Autodesk Fusion 360 part; units mm, degrees
(part 4 of 6)
  spline S229 degree 3 poles (64.9154, 36.2009) (64.8548, 36.2983) (64.7292, 36.5001) (64.6717, 36.7309) (64.642, 36.8503) knots 0 0 0 0 0.034206 0.07085 0.07085 0.07085 0.07085
  spline S230 degree 3 poles (64.642, 36.8503) (64.6279, 36.962) (64.5921, 37.2456) (64.5928, 37.5315) (64.5931, 37.7048) knots 0 0 0 0 0.033768 0.085663 0.085663 0.085663 0.085663
  line L165 (64.5931, 37.7048) -> (64.5931, 40.8932)
  line L166 (64.5931, 40.8932) -> (65.472, 40.8932)
  line L167 (65.472, 40.8932) -> (65.472, 37.7389)
  spline S231 degree 3 poles (65.472, 37.7389) (65.4729, 37.5814) (65.4743, 37.309) (65.5449, 37.0464) (65.5746, 36.9357) knots 0 0 0 0 0.047006 0.081267 0.081267 0.081267 0.081267
  spline S232 degree 3 poles (65.5746, 36.9357) (65.6162, 36.851) (65.7009, 36.6784) (65.8582, 36.5674) (65.9384, 36.5109) knots 0 0 0 0 0.027833 0.056732 0.056732 0.056732 0.056732
  spline S233 degree 3 poles (65.9384, 36.5109) (66.0312, 36.4646) (66.2241, 36.3686) (66.4395, 36.3578) (66.5511, 36.3522) knots 0 0 0 0 0.030776 0.063912 0.063912 0.063912 0.063912
  spline S234 degree 3 poles (66.5511, 36.3522) (66.7312, 36.3665) (67.0878, 36.3947) (67.3772, 36.6047) (67.5204, 36.7087) knots 0 0 0 0 0.053061 0.105073 0.105073 0.105073 0.105073
  spline S235 degree 3 poles (67.5204, 36.7087) (67.6385, 36.8753) (67.9223, 37.2758) (67.926, 37.7716) (67.9281, 38.0612) knots 0 0 0 0 0.060011 0.144248 0.144248 0.144248 0.144248
  line L168 (67.9281, 38.0612) -> (67.9281, 40.8932)
  line L169 (67.9281, 40.8932) -> (68.807, 40.8932)
  line L170 (56.9174, 39.2233) -> (56.0092, 39.3356)
  spline S236 degree 3 poles (56.0092, 39.3356) (56.0926, 39.5834) (56.2541, 40.0629) (56.6255, 40.4055) (56.8051, 40.571) knots 0 0 0 0 0.077034 0.149075 0.149075 0.149075 0.149075
  spline S237 degree 3 poles (56.8051, 40.571) (57.02, 40.699) (57.4764, 40.9709) (58.0081, 40.9968) (58.2894, 41.0104) knots 0 0 0 0 0.073917 0.156923 0.156923 0.156923 0.156923
  spline S238 degree 3 poles (58.2894, 41.0104) (58.6434, 40.987) (59.3202, 40.9421) (59.8438, 40.514) (60.0936, 40.3097) knots 0 0 0 0 0.103483 0.197891 0.197891 0.197891 0.197891
  spline S239 degree 3 poles (60.0936, 40.3097) (60.2877, 40.039) (60.7071, 39.454) (60.7416, 38.7321) (60.7601, 38.3444) knots 0 0 0 0 0.097893 0.211487 0.211487 0.211487 0.211487
  spline S240 degree 3 poles (60.7601, 38.3444) (60.7418, 37.9438) (60.7079, 37.2003) (60.2825, 36.5932) (60.0863, 36.3132) knots 0 0 0 0 0.117426 0.217964 0.217964 0.217964 0.217964
  spline S241 degree 3 poles (60.0863, 36.3132) (59.8409, 36.1024) (59.3383, 35.6707) (58.6768, 35.6177) (58.3383, 35.5905) knots 0 0 0 0 0.094484 0.193557 0.193557 0.193557 0.193557
  spline S242 degree 3 poles (58.3383, 35.5905) (58.0098, 35.6175) (57.3662, 35.6704) (56.8781, 36.092) (56.639, 36.2985) knots 0 0 0 0 0.096126 0.18838 0.18838 0.18838 0.18838
  spline S243 degree 3 poles (56.639, 36.2985) (56.4471, 36.5731) (56.0307, 37.1688) (55.9977, 37.8977) (55.9799, 38.2907) knots 0 0 0 0 0.098509 0.213708 0.213708 0.213708 0.213708
  spline S244 degree 3 poles (55.9799, 38.2907) (55.9802, 38.3233) (55.9809, 38.4014) (55.9833, 38.4795) (55.9847, 38.5251) knots 0 0 0 0 0.009766 0.023443 0.023443 0.023443 0.023443
  line L171 (55.9847, 38.5251) -> (59.8519, 38.5251)
  spline S245 degree 3 poles (59.8519, 38.5251) (59.8265, 38.7854) (59.7797, 39.2658) (59.4977, 39.6553) (59.3685, 39.8337) knots 0 0 0 0 0.076825 0.141746 0.141746 0.141746 0.141746
  spline S246 degree 3 poles (59.3685, 39.8337) (59.2137, 39.9661) (58.9013, 40.2335) (58.4914, 40.2696) (58.2845, 40.2878) knots 0 0 0 0 0.059532 0.120175 0.120175 0.120175 0.120175
  spline S247 degree 3 poles (58.2845, 40.2878) (58.1314, 40.2787) (57.8353, 40.2612) (57.5818, 40.1079) (57.4593, 40.0339) knots 0 0 0 0 0.045247 0.087501 0.087501 0.087501 0.087501
  spline S248 degree 3 poles (57.4593, 40.0339) (57.349, 39.9297) (57.1072, 39.7015) (56.9842, 39.3917) (56.9174, 39.2233) knots 0 0 0 0 0.045001 0.098557 0.098557 0.098557 0.098557
  line L172 (46.0238, 40.8932) -> (46.0238, 35.7077)
  line L173 (46.0238, 35.7077) -> (45.2328, 35.7077)
  line L174 (45.2328, 35.7077) -> (45.2328, 36.4938)
  spline S249 degree 3 poles (45.2328, 36.4938) (45.1447, 36.3341) (44.9948, 36.0624) (44.7674, 35.8527) (44.6737, 35.7663) knots 0 0 0 0 0.05425 0.092273 0.092273 0.092273 0.092273
  spline S250 degree 3 poles (44.6737, 35.7663) (44.5863, 35.715) (44.4119, 35.6128) (44.2103, 35.5979) (44.1097, 35.5905) knots 0 0 0 0 0.029972 0.059777 0.059777 0.059777 0.059777
  spline S251 degree 3 poles (44.1097, 35.5905) (43.9575, 35.6045) (43.6366, 35.6341) (43.3546, 35.7912) (43.2064, 35.8737) knots 0 0 0 0 0.045356 0.095599 0.095599 0.095599 0.095599
  line L175 (43.2064, 35.8737) -> (43.5092, 36.6891)
  spline S252 degree 3 poles (43.5092, 36.6891) (43.6143, 36.6336) (43.8166, 36.5268) (44.0443, 36.5078) (44.1537, 36.4987) knots 0 0 0 0 0.03525 0.067826 0.067826 0.067826 0.067826
  spline S253 degree 3 poles (44.1537, 36.4987) (44.2473, 36.5059) (44.4343, 36.5203) (44.5923, 36.6215) (44.6713, 36.672) knots 0 0 0 0 0.027685 0.055345 0.055345 0.055345 0.055345
  spline S254 degree 3 poles (44.6713, 36.672) (44.7427, 36.7369) (44.8902, 36.8708) (44.9616, 37.057) (44.9984, 37.153) knots 0 0 0 0 0.028537 0.058895 0.058895 0.058895 0.058895
  spline S255 degree 3 poles (44.9984, 37.153) (45.0411, 37.3157) (45.1294, 37.6518) (45.1396, 37.9992) (45.1449, 38.1784) knots 0 0 0 0 0.050287 0.103879 0.103879 0.103879 0.103879
  line L176 (45.1449, 38.1784) -> (45.1449, 40.8932)
  line L177 (45.1449, 40.8932) -> (46.0238, 40.8932)
  line L178 (42.6791, 40.8932) -> (42.6791, 35.7077)
  line L179 (42.6791, 35.7077) -> (41.8002, 35.7077)
  line L180 (41.8002, 35.7077) -> (41.8002, 40.8932)
  line L181 (41.8002, 40.8932) -> (42.6791, 40.8932)
  line L182 (40.8138, 39.3454) -> (39.9447, 39.2087)
  spline S256 degree 3 poles (39.9447, 39.2087) (39.9126, 39.3698) (39.8517, 39.6759) (39.6381, 39.9023) (39.537, 40.0095) knots 0 0 0 0 0.048178 0.091492 0.091492 0.091492 0.091492
  spline S257 degree 3 poles (39.537, 40.0095) (39.4069, 40.0905) (39.1219, 40.268) (38.785, 40.2808) (38.6019, 40.2878) knots 0 0 0 0 0.045208 0.099065 0.099065 0.099065 0.099065
  spline S258 degree 3 poles (38.6019, 40.2878) (38.4213, 40.2836) (38.0995, 40.2762) (37.8242, 40.1128) (37.7035, 40.0412) knots 0 0 0 0 0.053093 0.094556 0.094556 0.094556 0.094556
  spline S259 degree 3 poles (37.7035, 40.0412) (37.6181, 39.9579) (37.454, 39.7979) (37.4246, 39.5712) (37.4105, 39.4626) knots 0 0 0 0 0.034652 0.06657 0.06657 0.06657 0.06657
  spline S260 degree 3 poles (37.4105, 39.4626) (37.4218, 39.3682) (37.4447, 39.1773) (37.5938, 39.0555) (37.6693, 38.9938) knots 0 0 0 0 0.027386 0.055446 0.055446 0.055446 0.055446
  spline S261 degree 3 poles (37.6693, 38.9938) (37.7734, 38.9471) (38.0623, 38.8174) (38.3706, 38.7433) (38.5677, 38.696) knots 0 0 0 0 0.034189 0.094822 0.094822 0.094822 0.094822
  spline S262 degree 3 poles (38.5677, 38.696) (38.8428, 38.6271) (39.2983, 38.513) (39.7351, 38.3415) (39.9081, 38.2736) knots 0 0 0 0 0.084955 0.140654 0.140654 0.140654 0.140654
  spline S263 degree 3 poles (39.9081, 38.2736) (40.024, 38.2102) (40.2491, 38.0871) (40.4009, 37.8806) (40.4745, 37.7804) knots 0 0 0 0 0.039108 0.075916 0.075916 0.075916 0.075916
  spline S264 degree 3 poles (40.4745, 37.7804) (40.5307, 37.6722) (40.6442, 37.454) (40.6596, 37.2084) (40.6674, 37.0846) knots 0 0 0 0 0.036161 0.072917 0.072917 0.072917 0.072917
  spline S265 degree 3 poles (40.6674, 37.0846) (40.661, 36.9717) (40.6483, 36.7476) (40.5549, 36.5437) (40.5087, 36.4426) knots 0 0 0 0 0.033621 0.066662 0.066662 0.066662 0.066662
  spline S266 degree 3 poles (40.5087, 36.4426) (40.451, 36.3482) (40.3355, 36.1595) (40.1629, 36.0211) (40.0765, 35.9518) knots 0 0 0 0 0.032897 0.065829 0.065829 0.065829 0.065829
  spline S267 degree 3 poles (40.0765, 35.9518) (39.9973, 35.902) (39.8224, 35.792) (39.6253, 35.7296) (39.5175, 35.6955) knots 0 0 0 0 0.027973 0.061727 0.061727 0.061727 0.061727
  spline S268 degree 3 poles (39.5175, 35.6955) (39.3958, 35.6649) (39.1466, 35.6022) (38.8897, 35.5945) (38.7582, 35.5905) knots 0 0 0 0 0.037518 0.076851 0.076851 0.076851 0.076851
  spline S269 degree 3 poles (38.7582, 35.5905) (38.5656, 35.5961) (38.2002, 35.6067) (37.8514, 35.7151) (37.6864, 35.7663) knots 0 0 0 0 0.05748 0.109059 0.109059 0.109059 0.109059
  spline S270 degree 3 poles (37.6864, 35.7663) (37.546, 35.8258) (37.2846, 35.9365) (37.0936, 36.1456) (37.0052, 36.2424) knots 0 0 0 0 0.045124 0.083974 0.083974 0.083974 0.083974
  spline S271 degree 3 poles (37.0052, 36.2424) (36.9368, 36.3568) (36.7878, 36.6059) (36.7325, 36.8913) (36.7025, 37.0456) knots 0 0 0 0 0.039698 0.086419 0.086419 0.086419 0.086419
  line L183 (36.7025, 37.0456) -> (37.5619, 37.1628)
  spline S272 degree 3 poles (37.5619, 37.1628) (37.5891, 37.038) (37.6417, 36.7963) (37.8166, 36.622) (37.9012, 36.5378) knots 0 0 0 0 0.037427 0.072477 0.072477 0.072477 0.072477
  spline S273 degree 3 poles (37.9012, 36.5378) (38.0114, 36.4724) (38.2549, 36.3279) (38.5391, 36.3184) (38.6947, 36.3132) knots 0 0 0 0 0.037832 0.083649 0.083649 0.083649 0.083649
  spline S274 degree 3 poles (38.6947, 36.3132) (38.8716, 36.3146) (39.1763, 36.317) (39.4459, 36.4553) (39.559, 36.5134) knots 0 0 0 0 0.052121 0.089788 0.089788 0.089788 0.089788
  spline S275 degree 3 poles (39.559, 36.5134) (39.6344, 36.5801) (39.777, 36.7062) (39.8047, 36.8937) (39.8177, 36.9821) knots 0 0 0 0 0.029135 0.0551 0.0551 0.0551 0.0551
  spline S276 degree 3 poles (39.8177, 36.9821) (39.8132, 37.0378) (39.804, 37.1496) (39.7417, 37.2429) (39.7103, 37.2897) knots 0 0 0 0 0.016456 0.033067 0.033067 0.033067 0.033067
  spline S277 degree 3 poles (39.7103, 37.2897) (39.6666, 37.336) (39.5708, 37.4373) (39.4429, 37.4935) (39.3734, 37.5241) knots 0 0 0 0 0.018913 0.04141 0.04141 0.04141 0.04141
  spline S278 degree 3 poles (39.3734, 37.5241) (39.2869, 37.5514) (39.0299, 37.6324) (38.7696, 37.7023) (38.597, 37.7487) knots 0 0 0 0 0.027221 0.080828 0.080828 0.080828 0.080828
  spline S279 degree 3 poles (38.597, 37.7487) (38.3316, 37.8192) (37.8917, 37.936) (37.465, 38.0939) (37.2958, 38.1564) knots 0 0 0 0 0.082338 0.13643 0.13643 0.13643 0.13643
  spline S280 degree 3 poles (37.2958, 38.1564) (37.1803, 38.2141) (36.9546, 38.327) (36.7951, 38.5224) (36.7172, 38.6179) knots 0 0 0 0 0.038228 0.07476 0.07476 0.07476 0.07476
  spline S281 degree 3 poles (36.7172, 38.6179) (36.656, 38.7285) (36.5267, 38.962) (36.5139, 39.2292) (36.5072, 39.3698) knots 0 0 0 0 0.037411 0.079003 0.079003 0.079003 0.079003
  spline S282 degree 3 poles (36.5072, 39.3698) (36.5185, 39.5151) (36.5415, 39.8102) (36.6888, 40.0671) (36.7635, 40.1974) knots 0 0 0 0 0.043142 0.087613 0.087613 0.087613 0.087613
  spline S283 degree 3 poles (36.7635, 40.1974) (36.861, 40.3206) (37.0627, 40.5755) (37.3532, 40.7222) (37.5033, 40.798) knots 0 0 0 0 0.046534 0.096306 0.096306 0.096306 0.096306
  spline S284 degree 3 poles (37.5033, 40.798) (37.6733, 40.86) (38.0264, 40.9886) (38.4021, 41.003) (38.597, 41.0104) knots 0 0 0 0 0.053921 0.112025 0.112025 0.112025 0.112025
  spline S285 degree 3 poles (38.597, 41.0104) (38.9016, 41.0018) (39.4515, 40.9863) (39.9259, 40.7126) (40.1376, 40.5905) knots 0 0 0 0 0.089667 0.161897 0.161897 0.161897 0.161897
  spline S286 degree 3 poles (40.1376, 40.5905) (40.2994, 40.4263) (40.6433, 40.0773) (40.7548, 39.5988) (40.8138, 39.3454) knots 0 0 0 0 0.067824 0.14416 0.14416 0.14416 0.14416
  line L184 (42.6791, 34.7458) -> (42.6791, 33.735)
  line L185 (42.6791, 33.735) -> (41.8002, 33.735)
  line L186 (41.8002, 33.735) -> (41.8002, 34.7458)
  line L187 (41.8002, 34.7458) -> (42.6791, 34.7458)
  line L188 (51.5756, 42.8805) -> (51.5756, 35.7077)
  line L189 (51.5756, 35.7077) -> (50.7748, 35.7077)
  line L190 (50.7748, 35.7077) -> (50.7748, 36.3815)
  spline S287 degree 3 poles (50.7748, 36.3815) (50.6803, 36.2596) (50.4996, 36.0265) (50.2528, 35.8652) (50.1351, 35.7883) knots 0 0 0 0 0.045899 0.087785 0.087785 0.087785 0.087785
  spline S288 degree 3 poles (50.1351, 35.7883) (50.0056, 35.7306) (49.7309, 35.6084) (49.43, 35.5967) (49.2709, 35.5905) knots 0 0 0 0 0.042126 0.089382 0.089382 0.089382 0.089382
  spline S289 degree 3 poles (49.2709, 35.5905) (49.058, 35.6035) (48.6412, 35.6288) (48.2771, 35.8326) (48.099, 35.9323) knots 0 0 0 0 0.063081 0.123479 0.123479 0.123479 0.123479
  spline S290 degree 3 poles (48.099, 35.9323) (47.9391, 36.0605) (47.6107, 36.3236) (47.4268, 36.7024) (47.3324, 36.8967) knots 0 0 0 0 0.060684 0.124573 0.124573 0.124573 0.124573
  spline S291 degree 3 poles (47.3324, 36.8967) (47.2569, 37.1121) (47.1022, 37.5538) (47.0833, 38.0217) (47.0736, 38.2614) knots 0 0 0 0 0.068072 0.139594 0.139594 0.139594 0.139594
  spline S292 degree 3 poles (47.0736, 38.2614) (47.0838, 38.5162) (47.1036, 39.0093) (47.276, 39.4713) (47.3593, 39.6945) knots 0 0 0 0 0.075959 0.146956 0.146956 0.146956 0.146956
  spline S293 degree 3 poles (47.3593, 39.6945) (47.4631, 39.8932) (47.6662, 40.2816) (48.0176, 40.5432) (48.1893, 40.6711) knots 0 0 0 0 0.066289 0.129644 0.129644 0.129644 0.129644
  spline S294 degree 3 poles (48.1893, 40.6711) (48.3713, 40.77) (48.7291, 40.9646) (49.135, 40.9953) (49.3343, 41.0104) knots 0 0 0 0 0.061373 0.120639 0.120639 0.120639 0.120639
  spline S295 degree 3 poles (49.3343, 41.0104) (49.4754, 41.0036) (49.7498, 40.9903) (50.0009, 40.879) (50.1229, 40.8249) knots 0 0 0 0 0.041944 0.081634 0.081634 0.081634 0.081634
  spline S296 degree 3 poles (50.1229, 40.8249) (50.2332, 40.7601) (50.4488, 40.6335) (50.6153, 40.4471) (50.6967, 40.3561) knots 0 0 0 0 0.038106 0.074489 0.074489 0.074489 0.074489
  line L191 (50.6967, 40.3561) -> (50.6967, 42.8805)
  line L192 (50.6967, 42.8805) -> (51.5756, 42.8805)
  line L193 (27.483, 42.2234) -> (-5.7946, 42.2234) construction
  line L194 (-5.7946, 42.2234) -> (-5.7946, 34.7234) construction
  line L195 (-5.7946, 34.7234) -> (27.483, 34.7234) construction
  line L196 (27.483, 34.7234) -> (27.483, 42.2234) construction
  text T0 "Enterprise" font "Arial" height 7.5 align ink ink in box 0 x 0 at (27.483, 42.2234) x (-1, 0) y (0, -1) spacing 1 height is em
  constraint perpendicular L193 L194
  constraint parallel L193 L195
  constraint parallel L194 L196
extrude "Extrude22" add sketch "Sketch23" along normal blind 2 text T0 bodies 15
sketch "Sketch24" plane through (0, 3, 0) normal (0, 1, 0) x (-1, 0, 0)
  line L0 (27.473, 40.7129) -> (27.473, 35.3442)
  line L1 (27.473, 35.3442) -> (23.5912, 35.3442)
  line L2 (23.5912, 35.3442) -> (23.5912, 35.9778)
  line L3 (23.5912, 35.9778) -> (26.7626, 35.9778)
  line L4 (26.7626, 35.9778) -> (26.7626, 37.6221)
  line L5 (26.7626, 37.6221) -> (23.7926, 37.6221)
  line L6 (23.7926, 37.6221) -> (23.7926, 38.2519)
  line L7 (23.7926, 38.2519) -> (26.7626, 38.2519)
  line L8 (26.7626, 38.2519) -> (26.7626, 40.0793)
  line L9 (26.7626, 40.0793) -> (23.4667, 40.0793)
  line L10 (23.4667, 40.0793) -> (23.4667, 40.7129)
  line L11 (23.4667, 40.7129) -> (27.473, 40.7129)
  line L12 (16.9591, 40.1233) -> (16.8639, 40.7056)
  spline S0 degree 3 poles (16.8639, 40.7056) (16.9515, 40.7226) (17.1161, 40.7547) (17.2836, 40.7611) (17.3619, 40.7641) knots 0 0 0 0 0.026731 0.050214 0.050214 0.050214 0.050214
  spline S1 degree 3 poles (17.3619, 40.7641) (17.4698, 40.7621) (17.6628, 40.7584) (17.8403, 40.6836) (17.9186, 40.6506) knots 0 0 0 0 0.031987 0.057267 0.057267 0.057267 0.057267
  spline S2 degree 3 poles (17.9186, 40.6506) (17.9791, 40.6109) (18.0964, 40.534) (18.1641, 40.4114) (18.1969, 40.3522) knots 0 0 0 0 0.021363 0.04136 0.04136 0.04136 0.04136
  spline S3 degree 3 poles (18.1969, 40.3522) (18.2201, 40.2569) (18.282, 40.0018) (18.2792, 39.7387) (18.2775, 39.574) knots 0 0 0 0 0.029331 0.07849 0.07849 0.07849 0.07849
  line L13 (18.2775, 39.574) -> (18.2775, 37.3364)
  line L14 (18.2775, 37.3364) -> (18.7609, 37.3364)
  line L15 (18.7609, 37.3364) -> (18.7609, 36.8237)
  line L16 (18.7609, 36.8237) -> (18.2775, 36.8237)
  line L17 (18.2775, 36.8237) -> (18.2775, 35.8606)
  line L18 (18.2775, 35.8606) -> (17.622, 35.4651)
  line L19 (17.622, 35.4651) -> (17.622, 36.8237)
  line L20 (17.622, 36.8237) -> (16.9591, 36.8237)
  line L21 (16.9591, 36.8237) -> (16.9591, 37.3364)
  line L22 (16.9591, 37.3364) -> (17.622, 37.3364)
  line L23 (17.622, 37.3364) -> (17.622, 39.6106)
  spline S4 degree 3 poles (17.622, 39.6106) (17.6229, 39.6882) (17.6245, 39.8106) (17.5971, 39.9296) (17.5872, 39.9731) knots 0 0 0 0 0.023179 0.036529 0.036529 0.036529 0.036529
  spline S5 degree 3 poles (17.5872, 39.9731) (17.5736, 39.9987) (17.546, 40.0505) (17.498, 40.0842) (17.4736, 40.1013) knots 0 0 0 0 0.00856 0.01734 0.01734 0.01734 0.01734
  spline S6 degree 3 poles (17.4736, 40.1013) (17.4422, 40.1151) (17.3707, 40.1466) (17.2923, 40.1481) (17.2484, 40.1489) knots 0 0 0 0 0.010212 0.023221 0.023221 0.023221 0.023221
  spline S7 degree 3 poles (17.2484, 40.1489) (17.2059, 40.1474) (17.1091, 40.144) (17.013, 40.1307) (16.9591, 40.1233) knots 0 0 0 0 0.012742 0.02906 0.02906 0.02906 0.02906
  line L24 (12.1508, 40.7129) -> (12.1508, 36.8237)
  line L25 (12.1508, 36.8237) -> (11.5575, 36.8237)
  line L26 (11.5575, 36.8237) -> (11.5575, 37.4133)
  spline S8 degree 3 poles (11.5575, 37.4133) (11.4914, 37.2935) (11.379, 37.0898) (11.2085, 36.9325) (11.1382, 36.8677) knots 0 0 0 0 0.040688 0.069205 0.069205 0.069205 0.069205
  spline S9 degree 3 poles (11.1382, 36.8677) (11.0726, 36.8292) (10.9418, 36.7525) (10.7906, 36.7414) (10.7152, 36.7358) knots 0 0 0 0 0.022479 0.044833 0.044833 0.044833 0.044833
  spline S10 degree 3 poles (10.7152, 36.7358) (10.601, 36.7464) (10.3603, 36.7685) (10.1489, 36.8863) (10.0377, 36.9482) knots 0 0 0 0 0.034017 0.071699 0.071699 0.071699 0.071699
  line L27 (10.0377, 36.9482) -> (10.2648, 37.5598)
  spline S11 degree 3 poles (10.2648, 37.5598) (10.3436, 37.5182) (10.4953, 37.438) (10.6661, 37.4238) (10.7482, 37.417) knots 0 0 0 0 0.026437 0.050869 0.050869 0.050869 0.050869
  spline S12 degree 3 poles (10.7482, 37.417) (10.8184, 37.4224) (10.9586, 37.4332) (11.0771, 37.5091) (11.1364, 37.547) knots 0 0 0 0 0.020764 0.041509 0.041509 0.041509 0.041509
  spline S13 degree 3 poles (11.1364, 37.547) (11.19, 37.5956) (11.3006, 37.6961) (11.3541, 37.8357) (11.3817, 37.9077) knots 0 0 0 0 0.021403 0.044172 0.044172 0.044172 0.044172
  spline S14 degree 3 poles (11.3817, 37.9077) (11.4138, 38.0297) (11.4799, 38.2818) (11.4876, 38.5423) (11.4916, 38.6767) knots 0 0 0 0 0.037715 0.077909 0.077909 0.077909 0.077909
  line L28 (11.4916, 38.6767) -> (11.4916, 40.7129)
  line L29 (11.4916, 40.7129) -> (12.1508, 40.7129)
  line L30 (-5.1014, 39.4604) -> (-5.7826, 39.5447)
  spline S15 degree 3 poles (-5.7826, 39.5447) (-5.72, 39.7305) (-5.5989, 40.0901) (-5.3203, 40.347) (-5.1857, 40.4712) knots 0 0 0 0 0.057776 0.111807 0.111807 0.111807 0.111807
  spline S16 degree 3 poles (-5.1857, 40.4712) (-5.0244, 40.5672) (-4.6822, 40.7711) (-4.2833, 40.7905) (-4.0724, 40.8008) knots 0 0 0 0 0.055438 0.117692 0.117692 0.117692 0.117692
  spline S17 degree 3 poles (-4.0724, 40.8008) (-3.8069, 40.7832) (-3.2993, 40.7495) (-2.9066, 40.4284) (-2.7192, 40.2753) knots 0 0 0 0 0.077612 0.148419 0.148419 0.148419 0.148419
  spline S18 degree 3 poles (-2.7192, 40.2753) (-2.5736, 40.0722) (-2.2591, 39.6334) (-2.2333, 39.092) (-2.2194, 38.8013) knots 0 0 0 0 0.073419 0.158615 0.158615 0.158615 0.158615
  spline S19 degree 3 poles (-2.2194, 38.8013) (-2.2331, 38.5008) (-2.2585, 37.9432) (-2.5776, 37.4878) (-2.7247, 37.2778) knots 0 0 0 0 0.088069 0.163473 0.163473 0.163473 0.163473
  spline S20 degree 3 poles (-2.7247, 37.2778) (-2.9087, 37.1198) (-3.2857, 36.796) (-3.7818, 36.7562) (-4.0358, 36.7358) knots 0 0 0 0 0.070863 0.145168 0.145168 0.145168 0.145168
  spline S21 degree 3 poles (-4.0358, 36.7358) (-4.2821, 36.7561) (-4.7648, 36.7958) (-5.1309, 37.112) (-5.3102, 37.2668) knots 0 0 0 0 0.072095 0.141285 0.141285 0.141285 0.141285
  spline S22 degree 3 poles (-5.3102, 37.2668) (-5.4541, 37.4728) (-5.7665, 37.9195) (-5.7912, 38.4663) (-5.8046, 38.761) knots 0 0 0 0 0.073882 0.160281 0.160281 0.160281 0.160281
  spline S23 degree 3 poles (-5.8046, 38.761) (-5.8043, 38.7854) (-5.8038, 38.844) (-5.802, 38.9026) (-5.8009, 38.9368) knots 0 0 0 0 0.007325 0.017582 0.017582 0.017582 0.017582
  line L31 (-5.8009, 38.9368) -> (-2.9005, 38.9368)
  spline S24 degree 3 poles (-2.9005, 38.9368) (-2.9196, 39.132) (-2.9547, 39.4923) (-3.1662, 39.7844) (-3.2631, 39.9182) knots 0 0 0 0 0.057619 0.10631 0.10631 0.10631 0.10631
  spline S25 degree 3 poles (-3.2631, 39.9182) (-3.3791, 40.0175) (-3.6135, 40.218) (-3.9209, 40.2451) (-4.076, 40.2588) knots 0 0 0 0 0.044649 0.090131 0.090131 0.090131 0.090131
  spline S26 degree 3 poles (-4.076, 40.2588) (-4.1909, 40.252) (-4.413, 40.2389) (-4.6031, 40.1239) (-4.6949, 40.0683) knots 0 0 0 0 0.033935 0.065626 0.065626 0.065626 0.065626
  spline S27 degree 3 poles (-4.6949, 40.0683) (-4.7777, 39.9902) (-4.959, 39.8191) (-5.0513, 39.5867) (-5.1014, 39.4604) knots 0 0 0 0 0.033751 0.073918 0.073918 0.073918 0.073918
  line L32 (51.5756, 42.8805) -> (51.5756, 35.7077)
  line L33 (51.5756, 35.7077) -> (50.7748, 35.7077)
  line L34 (50.7748, 35.7077) -> (50.7748, 36.3815)
  spline S28 degree 3 poles (50.7748, 36.3815) (50.6803, 36.2596) (50.4996, 36.0265) (50.2528, 35.8652) (50.1351, 35.7883) knots 0 0 0 0 0.045899 0.087785 0.087785 0.087785 0.087785
  spline S29 degree 3 poles (50.1351, 35.7883) (50.0056, 35.7306) (49.7309, 35.6084) (49.43, 35.5967) (49.2709, 35.5905) knots 0 0 0 0 0.042126 0.089382 0.089382 0.089382 0.089382
  spline S30 degree 3 poles (49.2709, 35.5905) (49.058, 35.6035) (48.6412, 35.6288) (48.2771, 35.8326) (48.099, 35.9323) knots 0 0 0 0 0.063081 0.123479 0.123479 0.123479 0.123479
  spline S31 degree 3 poles (48.099, 35.9323) (47.9391, 36.0605) (47.6107, 36.3236) (47.4268, 36.7024) (47.3324, 36.8967) knots 0 0 0 0 0.060684 0.124573 0.124573 0.124573 0.124573
  spline S32 degree 3 poles (47.3324, 36.8967) (47.2569, 37.1121) (47.1022, 37.5538) (47.0833, 38.0217) (47.0736, 38.2614) knots 0 0 0 0 0.068072 0.139594 0.139594 0.139594 0.139594
  spline S33 degree 3 poles (47.0736, 38.2614) (47.0838, 38.5162) (47.1036, 39.0093) (47.276, 39.4713) (47.3593, 39.6945) knots 0 0 0 0 0.075959 0.146956 0.146956 0.146956 0.146956
  spline S34 degree 3 poles (47.3593, 39.6945) (47.4631, 39.8932) (47.6662, 40.2816) (48.0176, 40.5432) (48.1893, 40.6711) knots 0 0 0 0 0.066289 0.129644 0.129644 0.129644 0.129644
  spline S35 degree 3 poles (48.1893, 40.6711) (48.3713, 40.77) (48.7291, 40.9646) (49.135, 40.9953) (49.3343, 41.0104) knots 0 0 0 0 0.061373 0.120639 0.120639 0.120639 0.120639
  spline S36 degree 3 poles (49.3343, 41.0104) (49.4754, 41.0036) (49.7498, 40.9903) (50.0009, 40.879) (50.1229, 40.8249) knots 0 0 0 0 0.041944 0.081634 0.081634 0.081634 0.081634
  spline S37 degree 3 poles (50.1229, 40.8249) (50.2332, 40.7601) (50.4488, 40.6335) (50.6153, 40.4471) (50.6967, 40.3561) knots 0 0 0 0 0.038106 0.074489 0.074489 0.074489 0.074489
  line L35 (50.6967, 40.3561) -> (50.6967, 42.8805)
  line L36 (50.6967, 42.8805) -> (51.5756, 42.8805)
  line L37 (42.6791, 34.7458) -> (42.6791, 33.735)
  line L38 (42.6791, 33.735) -> (41.8002, 33.735)
  line L39 (41.8002, 33.735) -> (41.8002, 34.7458)
  line L40 (41.8002, 34.7458) -> (42.6791, 34.7458)
  line L41 (40.8138, 39.3454) -> (39.9447, 39.2087)
  spline S38 degree 3 poles (39.9447, 39.2087) (39.9126, 39.3698) (39.8517, 39.6759) (39.6381, 39.9023) (39.537, 40.0095) knots 0 0 0 0 0.048178 0.091492 0.091492 0.091492 0.091492
  spline S39 degree 3 poles (39.537, 40.0095) (39.4069, 40.0905) (39.1219, 40.268) (38.785, 40.2808) (38.6019, 40.2878) knots 0 0 0 0 0.045208 0.099065 0.099065 0.099065 0.099065
  spline S40 degree 3 poles (38.6019, 40.2878) (38.4213, 40.2836) (38.0995, 40.2762) (37.8242, 40.1128) (37.7035, 40.0412) knots 0 0 0 0 0.053093 0.094556 0.094556 0.094556 0.094556
  spline S41 degree 3 poles (37.7035, 40.0412) (37.6181, 39.9579) (37.454, 39.7979) (37.4246, 39.5712) (37.4105, 39.4626) knots 0 0 0 0 0.034652 0.06657 0.06657 0.06657 0.06657
  spline S42 degree 3 poles (37.4105, 39.4626) (37.4218, 39.3682) (37.4447, 39.1773) (37.5938, 39.0555) (37.6693, 38.9938) knots 0 0 0 0 0.027386 0.055446 0.055446 0.055446 0.055446
  spline S43 degree 3 poles (37.6693, 38.9938) (37.7734, 38.9471) (38.0623, 38.8174) (38.3706, 38.7433) (38.5677, 38.696) knots 0 0 0 0 0.034189 0.094822 0.094822 0.094822 0.094822
  spline S44 degree 3 poles (38.5677, 38.696) (38.8428, 38.6271) (39.2983, 38.513) (39.7351, 38.3415) (39.9081, 38.2736) knots 0 0 0 0 0.084955 0.140654 0.140654 0.140654 0.140654
  spline S45 degree 3 poles (39.9081, 38.2736) (40.024, 38.2102) (40.2491, 38.0871) (40.4009, 37.8806) (40.4745, 37.7804) knots 0 0 0 0 0.039108 0.075916 0.075916 0.075916 0.075916
  spline S46 degree 3 poles (40.4745, 37.7804) (40.5307, 37.6722) (40.6442, 37.454) (40.6596, 37.2084) (40.6674, 37.0846) knots 0 0 0 0 0.036161 0.072917 0.072917 0.072917 0.072917
  spline S47 degree 3 poles (40.6674, 37.0846) (40.661, 36.9717) (40.6483, 36.7476) (40.5549, 36.5437) (40.5087, 36.4426) knots 0 0 0 0 0.033621 0.066662 0.066662 0.066662 0.066662
  spline S48 degree 3 poles (40.5087, 36.4426) (40.451, 36.3482) (40.3355, 36.1595) (40.1629, 36.0211) (40.0765, 35.9518) knots 0 0 0 0 0.032897 0.065829 0.065829 0.065829 0.065829
  spline S49 degree 3 poles (40.0765, 35.9518) (39.9973, 35.902) (39.8224, 35.792) (39.6253, 35.7296) (39.5175, 35.6955) knots 0 0 0 0 0.027973 0.061727 0.061727 0.061727 0.061727
  spline S50 degree 3 poles (39.5175, 35.6955) (39.3958, 35.6649) (39.1466, 35.6022) (38.8897, 35.5945) (38.7582, 35.5905) knots 0 0 0 0 0.037518 0.076851 0.076851 0.076851 0.076851
  spline S51 degree 3 poles (38.7582, 35.5905) (38.5656, 35.5961) (38.2002, 35.6067) (37.8514, 35.7151) (37.6864, 35.7663) knots 0 0 0 0 0.05748 0.109059 0.109059 0.109059 0.109059
  spline S52 degree 3 poles (37.6864, 35.7663) (37.546, 35.8258) (37.2846, 35.9365) (37.0936, 36.1456) (37.0052, 36.2424) knots 0 0 0 0 0.045124 0.083974 0.083974 0.083974 0.083974
  spline S53 degree 3 poles (37.0052, 36.2424) (36.9368, 36.3568) (36.7878, 36.6059) (36.7325, 36.8913) (36.7025, 37.0456) knots 0 0 0 0 0.039698 0.086419 0.086419 0.086419 0.086419
  line L42 (36.7025, 37.0456) -> (37.5619, 37.1628)
  spline S54 degree 3 poles (37.5619, 37.1628) (37.5891, 37.038) (37.6417, 36.7963) (37.8166, 36.622) (37.9012, 36.5378) knots 0 0 0 0 0.037427 0.072477 0.072477 0.072477 0.072477
  spline S55 degree 3 poles (37.9012, 36.5378) (38.0114, 36.4724) (38.2549, 36.3279) (38.5391, 36.3184) (38.6947, 36.3132) knots 0 0 0 0 0.037832 0.083649 0.083649 0.083649 0.083649
  spline S56 degree 3 poles (38.6947, 36.3132) (38.8716, 36.3146) (39.1763, 36.317) (39.4459, 36.4553) (39.559, 36.5134) knots 0 0 0 0 0.052121 0.089788 0.089788 0.089788 0.089788
  spline S57 degree 3 poles (39.559, 36.5134) (39.6344, 36.5801) (39.777, 36.7062) (39.8047, 36.8937) (39.8177, 36.9821) knots 0 0 0 0 0.029135 0.0551 0.0551 0.0551 0.0551
  spline S58 degree 3 poles (39.8177, 36.9821) (39.8132, 37.0378) (39.804, 37.1496) (39.7417, 37.2429) (39.7103, 37.2897) knots 0 0 0 0 0.016456 0.033067 0.033067 0.033067 0.033067
  spline S59 degree 3 poles (39.7103, 37.2897) (39.6666, 37.336) (39.5708, 37.4373) (39.4429, 37.4935) (39.3734, 37.5241) knots 0 0 0 0 0.018913 0.04141 0.04141 0.04141 0.04141
  spline S60 degree 3 poles (39.3734, 37.5241) (39.2869, 37.5514) (39.0299, 37.6324) (38.7696, 37.7023) (38.597, 37.7487) knots 0 0 0 0 0.027221 0.080828 0.080828 0.080828 0.080828
  spline S61 degree 3 poles (38.597, 37.7487) (38.3316, 37.8192) (37.8917, 37.936) (37.465, 38.0939) (37.2958, 38.1564) knots 0 0 0 0 0.082338 0.13643 0.13643 0.13643 0.13643
  spline S62 degree 3 poles (37.2958, 38.1564) (37.1803, 38.2141) (36.9546, 38.327) (36.7951, 38.5224) (36.7172, 38.6179) knots 0 0 0 0 0.038228 0.07476 0.07476 0.07476 0.07476
  spline S63 degree 3 poles (36.7172, 38.6179) (36.656, 38.7285) (36.5267, 38.962) (36.5139, 39.2292) (36.5072, 39.3698) knots 0 0 0 0 0.037411 0.079003 0.079003 0.079003 0.079003
  spline S64 degree 3 poles (36.5072, 39.3698) (36.5185, 39.5151) (36.5415, 39.8102) (36.6888, 40.0671) (36.7635, 40.1974) knots 0 0 0 0 0.043142 0.087613 0.087613 0.087613 0.087613
  spline S65 degree 3 poles (36.7635, 40.1974) (36.861, 40.3206) (37.0627, 40.5755) (37.3532, 40.7222) (37.5033, 40.798) knots 0 0 0 0 0.046534 0.096306 0.096306 0.096306 0.096306
  spline S66 degree 3 poles (37.5033, 40.798) (37.6733, 40.86) (38.0264, 40.9886) (38.4021, 41.003) (38.597, 41.0104) knots 0 0 0 0 0.053921 0.112025 0.112025 0.112025 0.112025
  spline S67 degree 3 poles (38.597, 41.0104) (38.9016, 41.0018) (39.4515, 40.9863) (39.9259, 40.7126) (40.1376, 40.5905) knots 0 0 0 0 0.089667 0.161897 0.161897 0.161897 0.161897
  spline S68 degree 3 poles (40.1376, 40.5905) (40.2994, 40.4263) (40.6433, 40.0773) (40.7548, 39.5988) (40.8138, 39.3454) knots 0 0 0 0 0.067824 0.14416 0.14416 0.14416 0.14416
  line L43 (42.6791, 40.8932) -> (42.6791, 35.7077)
  line L44 (42.6791, 35.7077) -> (41.8002, 35.7077)
  line L45 (41.8002, 35.7077) -> (41.8002, 40.8932)
  line L46 (41.8002, 40.8932) -> (42.6791, 40.8932)
  line L47 (46.0238, 40.8932) -> (46.0238, 35.7077)
  line L48 (46.0238, 35.7077) -> (45.2328, 35.7077)
  line L49 (45.2328, 35.7077) -> (45.2328, 36.4938)
  spline S69 degree 3 poles (45.2328, 36.4938) (45.1447, 36.3341) (44.9948, 36.0624) (44.7674, 35.8527) (44.6737, 35.7663) knots 0 0 0 0 0.05425 0.092273 0.092273 0.092273 0.092273
  spline S70 degree 3 poles (44.6737, 35.7663) (44.5863, 35.715) (44.4119, 35.6128) (44.2103, 35.5979) (44.1097, 35.5905) knots 0 0 0 0 0.029972 0.059777 0.059777 0.059777 0.059777
  spline S71 degree 3 poles (44.1097, 35.5905) (43.9575, 35.6045) (43.6366, 35.6341) (43.3546, 35.7912) (43.2064, 35.8737) knots 0 0 0 0 0.045356 0.095599 0.095599 0.095599 0.095599
  line L50 (43.2064, 35.8737) -> (43.5092, 36.6891)
  spline S72 degree 3 poles (43.5092, 36.6891) (43.6143, 36.6336) (43.8166, 36.5268) (44.0443, 36.5078) (44.1537, 36.4987) knots 0 0 0 0 0.03525 0.067826 0.067826 0.067826 0.067826
  spline S73 degree 3 poles (44.1537, 36.4987) (44.2473, 36.5059) (44.4343, 36.5203) (44.5923, 36.6215) (44.6713, 36.672) knots 0 0 0 0 0.027685 0.055345 0.055345 0.055345 0.055345
  spline S74 degree 3 poles (44.6713, 36.672) (44.7427, 36.7369) (44.8902, 36.8708) (44.9616, 37.057) (44.9984, 37.153) knots 0 0 0 0 0.028537 0.058895 0.058895 0.058895 0.058895
  spline S75 degree 3 poles (44.9984, 37.153) (45.0411, 37.3157) (45.1294, 37.6518) (45.1396, 37.9992) (45.1449, 38.1784) knots 0 0 0 0 0.050287 0.103879 0.103879 0.103879 0.103879
  line L51 (45.1449, 38.1784) -> (45.1449, 40.8932)
  line L52 (45.1449, 40.8932) -> (46.0238, 40.8932)
  line L53 (56.9174, 39.2233) -> (56.0092, 39.3356)
  spline S76 degree 3 poles (56.0092, 39.3356) (56.0926, 39.5834) (56.2541, 40.0629) (56.6255, 40.4055) (56.8051, 40.571) knots 0 0 0 0 0.077034 0.149075 0.149075 0.149075 0.149075
  spline S77 degree 3 poles (56.8051, 40.571) (57.02, 40.699) (57.4764, 40.9709) (58.0081, 40.9968) (58.2894, 41.0104) knots 0 0 0 0 0.073917 0.156923 0.156923 0.156923 0.156923
  spline S78 degree 3 poles (58.2894, 41.0104) (58.6434, 40.987) (59.3202, 40.9421) (59.8438, 40.514) (60.0936, 40.3097) knots 0 0 0 0 0.103483 0.197891 0.197891 0.197891 0.197891
  spline S79 degree 3 poles (60.0936, 40.3097) (60.2877, 40.039) (60.7071, 39.454) (60.7416, 38.7321) (60.7601, 38.3444) knots 0 0 0 0 0.097893 0.211487 0.211487 0.211487 0.211487
  spline S80 degree 3 poles (60.7601, 38.3444) (60.7418, 37.9438) (60.7079, 37.2003) (60.2825, 36.5932) (60.0863, 36.3132) knots 0 0 0 0 0.117426 0.217964 0.217964 0.217964 0.217964
  spline S81 degree 3 poles (60.0863, 36.3132) (59.8409, 36.1024) (59.3383, 35.6707) (58.6768, 35.6177) (58.3383, 35.5905) knots 0 0 0 0 0.094484 0.193557 0.193557 0.193557 0.193557
  spline S82 degree 3 poles (58.3383, 35.5905) (58.0098, 35.6175) (57.3662, 35.6704) (56.8781, 36.092) (56.639, 36.2985) knots 0 0 0 0 0.096126 0.18838 0.18838 0.18838 0.18838
  spline S83 degree 3 poles (56.639, 36.2985) (56.4471, 36.5731) (56.0307, 37.1688) (55.9977, 37.8977) (55.9799, 38.2907) knots 0 0 0 0 0.098509 0.213708 0.213708 0.213708 0.213708
  spline S84 degree 3 poles (55.9799, 38.2907) (55.9802, 38.3233) (55.9809, 38.4014) (55.9833, 38.4795) (55.9847, 38.5251) knots 0 0 0 0 0.009766 0.023443 0.023443 0.023443 0.023443
  line L54 (55.9847, 38.5251) -> (59.8519, 38.5251)
  spline S85 degree 3 poles (59.8519, 38.5251) (59.8265, 38.7854) (59.7797, 39.2658) (59.4977, 39.6553) (59.3685, 39.8337) knots 0 0 0 0 0.076825 0.141746 0.141746 0.141746 0.141746
  spline S86 degree 3 poles (59.3685, 39.8337) (59.2137, 39.9661) (58.9013, 40.2335) (58.4914, 40.2696) (58.2845, 40.2878) knots 0 0 0 0 0.059532 0.120175 0.120175 0.120175 0.120175
  spline S87 degree 3 poles (58.2845, 40.2878) (58.1314, 40.2787) (57.8353, 40.2612) (57.5818, 40.1079) (57.4593, 40.0339) knots 0 0 0 0 0.045247 0.087501 0.087501 0.087501 0.087501
  spline S88 degree 3 poles (57.4593, 40.0339) (57.349, 39.9297) (57.1072, 39.7015) (56.9842, 39.3917) (56.9174, 39.2233) knots 0 0 0 0 0.045001 0.098557 0.098557 0.098557 0.098557
  line L55 (68.807, 40.8932) -> (68.807, 35.7077)
  line L56 (68.807, 35.7077) -> (68.016, 35.7077)
  line L57 (68.016, 35.7077) -> (68.016, 36.445)
  spline S89 degree 3 poles (68.016, 36.445) (67.8018, 36.1958) (67.3672, 35.69) (66.7027, 35.624) (66.3656, 35.5905) knots 0 0 0 0 0.094776 0.192358 0.192358 0.192358 0.192358
  spline S90 degree 3 poles (66.3656, 35.5905) (66.2141, 35.5968) (65.9182, 35.6092) (65.6397, 35.7098) (65.5038, 35.759) knots 0 0 0 0 0.04518 0.088272 0.088272 0.088272 0.088272
  spline S91 degree 3 poles (65.5038, 35.759) (65.3834, 35.8162) (65.157, 35.924) (64.9925, 36.1126) (64.9154, 36.2009) knots 0 0 0 0 0.039495 0.074282 0.074282 0.074282 0.074282
  spline S92 degree 3 poles (64.9154, 36.2009) (64.8548, 36.2983) (64.7292, 36.5001) (64.6717, 36.7309) (64.642, 36.8503) knots 0 0 0 0 0.034206 0.07085 0.07085 0.07085 0.07085
  spline S93 degree 3 poles (64.642, 36.8503) (64.6279, 36.962) (64.5921, 37.2456) (64.5928, 37.5315) (64.5931, 37.7048) knots 0 0 0 0 0.033768 0.085663 0.085663 0.085663 0.085663
  line L58 (64.5931, 37.7048) -> (64.5931, 40.8932)
  line L59 (64.5931, 40.8932) -> (65.472, 40.8932)
  line L60 (65.472, 40.8932) -> (65.472, 37.7389)
  spline S94 degree 3 poles (65.472, 37.7389) (65.4729, 37.5814) (65.4743, 37.309) (65.5449, 37.0464) (65.5746, 36.9357) knots 0 0 0 0 0.047006 0.081267 0.081267 0.081267 0.081267
  spline S95 degree 3 poles (65.5746, 36.9357) (65.6162, 36.851) (65.7009, 36.6784) (65.8582, 36.5674) (65.9384, 36.5109) knots 0 0 0 0 0.027833 0.056732 0.056732 0.056732 0.056732
  spline S96 degree 3 poles (65.9384, 36.5109) (66.0312, 36.4646) (66.2241, 36.3686) (66.4395, 36.3578) (66.5511, 36.3522) knots 0 0 0 0 0.030776 0.063912 0.063912 0.063912 0.063912
  spline S97 degree 3 poles (66.5511, 36.3522) (66.7312, 36.3665) (67.0878, 36.3947) (67.3772, 36.6047) (67.5204, 36.7087) knots 0 0 0 0 0.053061 0.105073 0.105073 0.105073 0.105073
  spline S98 degree 3 poles (67.5204, 36.7087) (67.6385, 36.8753) (67.9223, 37.2758) (67.926, 37.7716) (67.9281, 38.0612) knots 0 0 0 0 0.060011 0.144248 0.144248 0.144248 0.144248
  line L61 (67.9281, 38.0612) -> (67.9281, 40.8932)
  line L62 (67.9281, 40.8932) -> (68.807, 40.8932)
  line L63 (74.99, 55.7007) -> (74.99, 44.9634)
  line L64 (74.99, 44.9634) -> (67.2263, 44.9634)
  line L65 (67.2263, 44.9634) -> (67.2263, 46.2305)
  line L66 (67.2263, 46.2305) -> (73.5691, 46.2305)
  line L67 (73.5691, 46.2305) -> (73.5691, 49.519)
  line L68 (73.5691, 49.519) -> (67.6292, 49.519)
  line L69 (67.6292, 49.519) -> (67.6292, 50.7788)
  line L70 (67.6292, 50.7788) -> (73.5691, 50.7788)
  line L71 (73.5691, 50.7788) -> (73.5691, 54.4336)
  line L72 (73.5691, 54.4336) -> (66.9773, 54.4336)
  line L73 (66.9773, 54.4336) -> (66.9773, 55.7007)
  line L74 (66.9773, 55.7007) -> (74.99, 55.7007)
  line L75 (53.9622, 54.5215) -> (53.7717, 55.686)
  spline S99 degree 3 poles (53.7717, 55.686) (53.947, 55.7202) (54.2761, 55.7843) (54.6112, 55.7972) (54.7678, 55.8032) knots 0 0 0 0 0.053462 0.100428 0.100428 0.100428 0.100428
  spline S100 degree 3 poles (54.7678, 55.8032) (54.9835, 55.7991) (55.3696, 55.7916) (55.7244, 55.6422) (55.8811, 55.5762) knots 0 0 0 0 0.063973 0.114534 0.114534 0.114534 0.114534
  spline S101 degree 3 poles (55.8811, 55.5762) (56.0022, 55.4967) (56.2367, 55.3428) (56.3722, 55.0977) (56.4378, 54.9792) knots 0 0 0 0 0.042726 0.08272 0.08272 0.08272 0.08272
  spline S102 degree 3 poles (56.4378, 54.9792) (56.4841, 54.7887) (56.608, 54.2786) (56.6024, 53.7524) (56.5989, 53.4228) knots 0 0 0 0 0.058662 0.156981 0.156981 0.156981 0.156981
  line L76 (56.5989, 53.4228) -> (56.5989, 48.9478)
  line L77 (56.5989, 48.9478) -> (57.5657, 48.9478)
  line L78 (57.5657, 48.9478) -> (57.5657, 47.9224)
  line L79 (57.5657, 47.9224) -> (56.5989, 47.9224)
  line L80 (56.5989, 47.9224) -> (56.5989, 45.9961)
  line L81 (56.5989, 45.9961) -> (55.2879, 45.2051)
  line L82 (55.2879, 45.2051) -> (55.2879, 47.9224)
  line L83 (55.2879, 47.9224) -> (53.9622, 47.9224)
  line L84 (53.9622, 47.9224) -> (53.9622, 48.9478)
  line L85 (53.9622, 48.9478) -> (55.2879, 48.9478)
  line L86 (55.2879, 48.9478) -> (55.2879, 53.4961)
  spline S103 degree 3 poles (55.2879, 53.4961) (55.2898, 53.6514) (55.2929, 53.8962) (55.2382, 54.1342) (55.2183, 54.2212) knots 0 0 0 0 0.046358 0.073057 0.073057 0.073057 0.073057
  spline S104 degree 3 poles (55.2183, 54.2212) (55.1911, 54.2723) (55.136, 54.376) (55.0399, 54.4434) (54.9912, 54.4775) knots 0 0 0 0 0.017119 0.034679 0.034679 0.034679 0.034679
  spline S105 degree 3 poles (54.9912, 54.4775) (54.9283, 54.5052) (54.7853, 54.5681) (54.6286, 54.5711) (54.5408, 54.5728) knots 0 0 0 0 0.020424 0.046442 0.046442 0.046442 0.046442
  spline S106 degree 3 poles (54.5408, 54.5728) (54.4558, 54.5697) (54.2621, 54.5629) (54.07, 54.5364) (53.9622, 54.5215) knots 0 0 0 0 0.025484 0.058121 0.058121 0.058121 0.058121
  line L87 (44.3455, 55.7007) -> (44.3455, 47.9224)
  line L88 (44.3455, 47.9224) -> (43.1589, 47.9224)
  line L89 (43.1589, 47.9224) -> (43.1589, 49.1016)
  spline S107 degree 3 poles (43.1589, 49.1016) (43.0268, 48.862) (42.802, 48.4545) (42.4609, 48.1399) (42.3203, 48.0103) knots 0 0 0 0 0.081375 0.138409 0.138409 0.138409 0.138409
  spline S108 degree 3 poles (42.3203, 48.0103) (42.1892, 47.9333) (41.9276, 47.78) (41.6252, 47.7577) (41.4744, 47.7466) knots 0 0 0 0 0.044958 0.089666 0.089666 0.089666 0.089666
  spline S109 degree 3 poles (41.4744, 47.7466) (41.246, 47.7676) (40.7646, 47.812) (40.3417, 48.0476) (40.1194, 48.1714) knots 0 0 0 0 0.068034 0.143398 0.143398 0.143398 0.143398
  line L90 (40.1194, 48.1714) -> (40.5735, 49.3945)
  spline S110 degree 3 poles (40.5735, 49.3945) (40.7312, 49.3113) (41.0346, 49.151) (41.3762, 49.1226) (41.5403, 49.1089) knots 0 0 0 0 0.052874 0.101739 0.101739 0.101739 0.101739
  spline S111 degree 3 poles (41.5403, 49.1089) (41.6806, 49.1197) (41.9612, 49.1413) (42.1982, 49.2931) (42.3167, 49.3689) knots 0 0 0 0 0.041528 0.083017 0.083017 0.083017 0.083017
  spline S112 degree 3 poles (42.3167, 49.3689) (42.4239, 49.4662) (42.6451, 49.667) (42.7522, 49.9464) (42.8074, 50.0903) knots 0 0 0 0 0.042806 0.088343 0.088343 0.088343 0.088343
  spline S113 degree 3 poles (42.8074, 50.0903) (42.8715, 50.3344) (43.0038, 50.8385) (43.0192, 51.3596) (43.0271, 51.6284) knots 0 0 0 0 0.075431 0.155819 0.155819 0.155819 0.155819
  line L91 (43.0271, 51.6284) -> (43.0271, 55.7007)
  line L92 (43.0271, 55.7007) -> (44.3455, 55.7007)
  line L93 (9.8411, 53.1958) -> (8.4788, 53.3643)
  spline S114 degree 3 poles (8.4788, 53.3643) (8.6039, 53.7359) (8.8461, 54.4552) (9.4033, 54.969) (9.6726, 55.2173) knots 0 0 0 0 0.115551 0.223613 0.223613 0.223613 0.223613
  spline S115 degree 3 poles (9.6726, 55.2173) (9.9951, 55.4094) (10.6796, 55.8172) (11.4773, 55.8559) (11.8992, 55.8765) knots 0 0 0 0 0.110875 0.235384 0.235384 0.235384 0.235384
  spline S116 degree 3 poles (11.8992, 55.8765) (12.4301, 55.8413) (13.4453, 55.774) (14.2308, 55.1318) (14.6055, 54.8254) knots 0 0 0 0 0.155225 0.296837 0.296837 0.296837 0.296837
  spline S117 degree 3 poles (14.6055, 54.8254) (14.8966, 54.4193) (15.5257, 53.5417) (15.5774, 52.459) (15.6052, 51.8774) knots 0 0 0 0 0.146839 0.31723 0.31723 0.31723 0.31723
  spline S118 degree 3 poles (15.6052, 51.8774) (15.5778, 51.2766) (15.5269, 50.1613) (14.8888, 49.2506) (14.5945, 48.8306) knots 0 0 0 0 0.176138 0.326947 0.326947 0.326947 0.326947
  spline S119 degree 3 poles (14.5945, 48.8306) (14.2265, 48.5145) (13.4725, 47.8669) (12.4803, 47.7873) (11.9724, 47.7466) knots 0 0 0 0 0.141726 0.290335 0.290335 0.290335 0.290335
  spline S120 degree 3 poles (11.9724, 47.7466) (11.4798, 47.7871) (10.5143, 47.8664) (9.7821, 48.4989) (9.4236, 48.8086) knots 0 0 0 0 0.144189 0.28257 0.28257 0.28257 0.28257
  spline S121 degree 3 poles (9.4236, 48.8086) (9.1357, 49.2205) (8.511, 50.114) (8.4615, 51.2074) (8.4348, 51.7969) knots 0 0 0 0 0.147764 0.320562 0.320562 0.320562 0.320562
  spline S122 degree 3 poles (8.4348, 51.7969) (8.4353, 51.8457) (8.4364, 51.9629) (8.44, 52.0801) (8.4421, 52.1484) knots 0 0 0 0 0.01465 0.035165 0.035165 0.035165 0.035165
  line L94 (8.4421, 52.1484) -> (14.2429, 52.1484)
  spline S123 degree 3 poles (14.2429, 52.1484) (14.2048, 52.539) (14.1345, 53.2596) (13.7116, 53.8438) (13.5178, 54.1113) knots 0 0 0 0 0.115238 0.212619 0.212619 0.212619 0.212619
  spline S124 degree 3 poles (13.5178, 54.1113) (13.2856, 54.31) (12.8169, 54.711) (12.2021, 54.7652) (11.8919, 54.7925) knots 0 0 0 0 0.089299 0.180262 0.180262 0.180262 0.180262
  spline S125 degree 3 poles (11.8919, 54.7925) (11.6622, 54.7789) (11.218, 54.7526) (10.8377, 54.5227) (10.6541, 54.4116) knots 0 0 0 0 0.067871 0.131252 0.131252 0.131252 0.131252
  spline S126 degree 3 poles (10.6541, 54.4116) (10.4885, 54.2553) (10.1259, 53.913) (9.9413, 53.4483) (9.8411, 53.1958) knots 0 0 0 0 0.067501 0.147835 0.147835 0.147835 0.147835
  line L95 (29.7082, 78.5459) -> (29.7082, 64.2002)
  line L96 (29.7082, 64.2002) -> (28.1067, 64.2002)
  line L97 (28.1067, 64.2002) -> (28.1067, 65.5478)
  spline S127 degree 3 poles (28.1067, 65.5478) (27.9177, 65.304) (27.5563, 64.8377) (27.0628, 64.5152) (26.8274, 64.3613) knots 0 0 0 0 0.091799 0.17557 0.17557 0.17557 0.17557
  spline S128 degree 3 poles (26.8274, 64.3613) (26.5684, 64.246) (26.0189, 64.0015) (25.4171, 63.9781) (25.0989, 63.9658) knots 0 0 0 0 0.084252 0.178765 0.178765 0.178765 0.178765
  spline S129 degree 3 poles (25.0989, 63.9658) (24.673, 63.9917) (23.8395, 64.0425) (23.1113, 64.45) (22.7551, 64.6494) knots 0 0 0 0 0.126163 0.246958 0.246958 0.246958 0.246958
  spline S130 degree 3 poles (22.7551, 64.6494) (22.4352, 64.9057) (21.7786, 65.432) (21.4106, 66.1896) (21.2219, 66.5781) knots 0 0 0 0 0.121368 0.249146 0.249146 0.249146 0.249146
  spline S131 degree 3 poles (21.2219, 66.5781) (21.071, 67.0089) (20.7615, 67.8924) (20.7237, 68.8282) (20.7043, 69.3076) knots 0 0 0 0 0.136145 0.279187 0.279187 0.279187 0.279187
  spline S132 degree 3 poles (20.7043, 69.3076) (20.7248, 69.8173) (20.7643, 70.8033) (21.109, 71.7274) (21.2756, 72.1738) knots 0 0 0 0 0.151918 0.293913 0.293913 0.293913 0.293913
  spline S133 degree 3 poles (21.2756, 72.1738) (21.4833, 72.5711) (21.8896, 73.3481) (22.5923, 73.8712) (22.9358, 74.1269) knots 0 0 0 0 0.132578 0.259289 0.259289 0.259289 0.259289
  spline S134 degree 3 poles (22.9358, 74.1269) (23.2998, 74.3249) (24.0153, 74.7139) (24.827, 74.7754) (25.2258, 74.8056) knots 0 0 0 0 0.122747 0.241277 0.241277 0.241277 0.241277
  spline S135 degree 3 poles (25.2258, 74.8056) (25.5078, 74.792) (26.0568, 74.7653) (26.5588, 74.5428) (26.803, 74.4345) knots 0 0 0 0 0.083889 0.163269 0.163269 0.163269 0.163269
  spline S136 degree 3 poles (26.803, 74.4345) (27.0235, 74.305) (27.4546, 74.0517) (27.7877, 73.6791) (27.9504, 73.497) knots 0 0 0 0 0.076211 0.148977 0.148977 0.148977 0.148977
  line L98 (27.9504, 73.497) -> (27.9504, 78.5459)
  line L99 (27.9504, 78.5459) -> (29.7082, 78.5459)
  line L100 (11.9153, 62.2763) -> (11.9153, 60.2549)
  line L101 (11.9153, 60.2549) -> (10.1575, 60.2549)
  line L102 (10.1575, 60.2549) -> (10.1575, 62.2763)
  line L103 (10.1575, 62.2763) -> (11.9153, 62.2763)
  line L104 (8.1848, 71.4756) -> (6.4465, 71.2021)
  spline S137 degree 3 poles (6.4465, 71.2021) (6.3824, 71.5245) (6.2606, 72.1366) (5.8334, 72.5894) (5.6311, 72.8037) knots 0 0 0 0 0.096356 0.182984 0.182984 0.182984 0.182984
  spline S138 degree 3 poles (5.6311, 72.8037) (5.3709, 72.9657) (4.8009, 73.3208) (4.1272, 73.3464) (3.761, 73.3603) knots 0 0 0 0 0.090416 0.19813 0.19813 0.19813 0.19813
  spline S139 degree 3 poles (3.761, 73.3603) (3.3996, 73.352) (2.7562, 73.3372) (2.2055, 73.0104) (1.9641, 72.8672) knots 0 0 0 0 0.106187 0.189111 0.189111 0.189111 0.189111
  spline S140 degree 3 poles (1.9641, 72.8672) (1.7933, 72.7006) (1.4651, 72.3805) (1.4063, 71.9272) (1.3782, 71.7099) knots 0 0 0 0 0.069303 0.133141 0.133141 0.133141 0.133141
  spline S141 degree 3 poles (1.3782, 71.7099) (1.4008, 71.5213) (1.4465, 71.1393) (1.7448, 70.8957) (1.8957, 70.7724) knots 0 0 0 0 0.054773 0.110892 0.110892 0.110892 0.110892
  spline S142 degree 3 poles (1.8957, 70.7724) (2.104, 70.6789) (2.6816, 70.4195) (3.2983, 70.2714) (3.6926, 70.1767) knots 0 0 0 0 0.068379 0.189643 0.189643 0.189643 0.189643
  spline S143 degree 3 poles (3.6926, 70.1767) (4.2428, 70.0389) (5.1537, 69.8107) (6.0273, 69.4678) (6.3733, 69.332) knots 0 0 0 0 0.169911 0.281309 0.281309 0.281309 0.281309
  spline S144 degree 3 poles (6.3733, 69.332) (6.6051, 69.2051) (7.0553, 68.9589) (7.3589, 68.5459) (7.5061, 68.3457) knots 0 0 0 0 0.078215 0.151833 0.151833 0.151833 0.151833
  spline S145 degree 3 poles (7.5061, 68.3457) (7.6186, 68.1292) (7.8455, 67.6927) (7.8763, 67.2016) (7.8918, 66.9541) knots 0 0 0 0 0.072323 0.145834 0.145834 0.145834 0.145834
  spline S146 degree 3 poles (7.8918, 66.9541) (7.8791, 66.7281) (7.8538, 66.28) (7.667, 65.8721) (7.5744, 65.6699) knots 0 0 0 0 0.067242 0.133324 0.133324 0.133324 0.133324
  spline S147 degree 3 poles (7.5744, 65.6699) (7.459, 65.4813) (7.2281, 65.1038) (6.8829, 64.8269) (6.7102, 64.6884) knots 0 0 0 0 0.065793 0.131657 0.131657 0.131657 0.131657
  spline S148 degree 3 poles (6.7102, 64.6884) (6.5517, 64.5887) (6.202, 64.3687) (5.8077, 64.244) (5.592, 64.1757) knots 0 0 0 0 0.055946 0.123455 0.123455 0.123455 0.123455
  spline S149 degree 3 poles (5.592, 64.1757) (5.3487, 64.1145) (4.8503, 63.9891) (4.3365, 63.9737) (4.0735, 63.9658) knots 0 0 0 0 0.075035 0.153702 0.153702 0.153702 0.153702
  spline S150 degree 3 poles (4.0735, 63.9658) (3.6883, 63.977) (2.9576, 63.9983) (2.2599, 64.2149) (1.9299, 64.3174) knots 0 0 0 0 0.11496 0.218119 0.218119 0.218119 0.218119
  spline S151 degree 3 poles (1.9299, 64.3174) (1.649, 64.4364) (1.1263, 64.6578) (0.7443, 65.076) (0.5676, 65.2695) knots 0 0 0 0 0.090247 0.167948 0.167948 0.167948 0.167948
  spline S152 degree 3 poles (0.5676, 65.2695) (0.4307, 65.4984) (0.1328, 65.9966) (0.022, 66.5674) (-0.0379, 66.8759) knots 0 0 0 0 0.079396 0.172838 0.172838 0.172838 0.172838
  line L105 (-0.0379, 66.8759) -> (1.6809, 67.1103)
  spline S153 degree 3 poles (1.6809, 67.1103) (1.7352, 66.8607) (1.8405, 66.3773) (2.1904, 66.0288) (2.3596, 65.8603) knots 0 0 0 0 0.074855 0.144953 0.144953 0.144953 0.144953
  spline S154 degree 3 poles (2.3596, 65.8603) (2.5799, 65.7296) (3.067, 65.4406) (3.6353, 65.4215) (3.9465, 65.4111) knots 0 0 0 0 0.075664 0.167297 0.167297 0.167297 0.167297
  spline S155 degree 3 poles (3.9465, 65.4111) (4.3003, 65.414) (4.9097, 65.4189) (5.4488, 65.6955) (5.675, 65.8115) knots 0 0 0 0 0.104241 0.179577 0.179577 0.179577 0.179577
  spline S156 degree 3 poles (5.675, 65.8115) (5.8258, 65.9449) (6.1111, 66.1972) (6.1665, 66.5723) (6.1926, 66.749) knots 0 0 0 0 0.05827 0.110201 0.110201 0.110201 0.110201
  spline S157 degree 3 poles (6.1926, 66.749) (6.1835, 66.8603) (6.1652, 67.0839) (6.0404, 67.2705) (5.9778, 67.3642) knots 0 0 0 0 0.032912 0.066134 0.066134 0.066134 0.066134
  spline S158 degree 3 poles (5.9778, 67.3642) (5.8903, 67.4568) (5.6987, 67.6593) (5.4429, 67.7719) (5.3039, 67.833) knots 0 0 0 0 0.037826 0.08282 0.08282 0.08282 0.08282
  spline S159 degree 3 poles (5.3039, 67.833) (5.1308, 67.8875) (4.6169, 68.0495) (4.0964, 68.1894) (3.7512, 68.2822) knots 0 0 0 0 0.054441 0.161656 0.161656 0.161656 0.161656
  spline S160 degree 3 poles (3.7512, 68.2822) (3.2203, 68.4232) (2.3405, 68.6568) (1.4871, 68.9725) (1.1487, 69.0976) knots 0 0 0 0 0.164675 0.27286 0.27286 0.27286 0.27286
  spline S161 degree 3 poles (1.1487, 69.0976) (0.9178, 69.213) (0.4663, 69.4388) (0.1473, 69.8295) (-0.0086, 70.0205) knots 0 0 0 0 0.076456 0.14952 0.14952 0.14952 0.14952
  spline S162 degree 3 poles (-0.0086, 70.0205) (-0.1309, 70.2417) (-0.3894, 70.7089) (-0.415, 71.2431) (-0.4285, 71.5244) knots 0 0 0 0 0.074822 0.158007 0.158007 0.158007 0.158007
  spline S163 degree 3 poles (-0.4285, 71.5244) (-0.4059, 71.815) (-0.3599, 72.4051) (-0.0653, 72.9189) (0.0842, 73.1797) knots 0 0 0 0 0.086284 0.175226 0.175226 0.175226 0.175226
  spline S164 degree 3 poles (0.0842, 73.1797) (0.2791, 73.426) (0.6826, 73.9358) (1.2635, 74.2292) (1.5637, 74.3808) knots 0 0 0 0 0.093067 0.192613 0.192613 0.192613 0.192613
  spline S165 degree 3 poles (1.5637, 74.3808) (1.9036, 74.5047) (2.6099, 74.762) (3.3614, 74.7907) (3.7512, 74.8056) knots 0 0 0 0 0.107841 0.22405 0.22405 0.22405 0.22405
  spline S166 degree 3 poles (3.7512, 74.8056) (4.3603, 74.7884) (5.46, 74.7574) (6.4089, 74.21) (6.8323, 73.9658) knots 0 0 0 0 0.179334 0.323794 0.323794 0.323794 0.323794